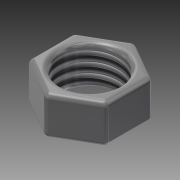
# Autodesk Inventor part: 3MNut
Saved by Autodesk Inventor 2015 (Build 190159000, 159)
## iProperties
Created: 2018-03-01
Part Number: 3MNut
Material: Stainless Steel
Document SubType Name: Modeling
Designer: Silas
Density: 8 g/cm^3
Appearance: Semi-Polished
Author: Silas
Autodesk Inventor part; units mm, degrees
ref_plane "YZ Plane" through (0, 0, 0) normal (1, 0, 0) x (0, 1, 0)
ref_plane "XZ Plane" through (0, 0, 0) normal (0, 1, 0) x (-1, 0, 0)
ref_plane "XY Plane" through (0, 0, 0) normal (0, 0, 1) x (1, 0, 0)
sketch "Sketch1" plane through (0, 0, 0) normal (0, 0, 1) x (1, 0, 0)
  circle A0 centre (0, 0) radius 1.5
  line L0 (0, 2.3094) -> (2, 1.1547)
  line L1 (2, 1.1547) -> (2, -1.1547)
  line L2 (2, -1.1547) -> (0, -2.3094)
  line L3 (0, -2.3094) -> (-2, -1.1547)
  line L4 (-2, -1.1547) -> (-2, 1.1547)
  line L5 (-2, 1.1547) -> (0, 2.3094)
  dimension "d0" = 3
  dimension "d1" = 2
  constraints: 12 end point, 2 coincident, 1 centre point, 13 other
  measures "d0" diameter of A0
  measures "d1" distance from line of point (0, 0) L1
extrude "Extrusion1" add sketch "Sketch1" along normal blind 2
thread "Thread1" size "M3x0.5" class "6H" standard "ANSI Metric M Profile" full length
fillet "Fillet1" radius 0.25 20 edges at (1, 1.7321, 2) (-1.5, 0, 2) (2, 0, 2) (1, -1.7321, 2) (-1.5, 0, 0) (-1, 1.7321, 2) (-2, 0, 2) (-1, -1.7321, 2) (2, 0, 0) (1, 1.7321, 0) (-1, 1.7321, 0) (-2, 0, 0) (-1, -1.7321, 0) (1, -1.7321, 0) (0, 2.3094, 1) (2, 1.1547, 1) (2, -1.1547, 1) (0, -2.3094, 1) (-2, -1.1547, 1) (-2, 1.1547, 1)
body "Solid1"
